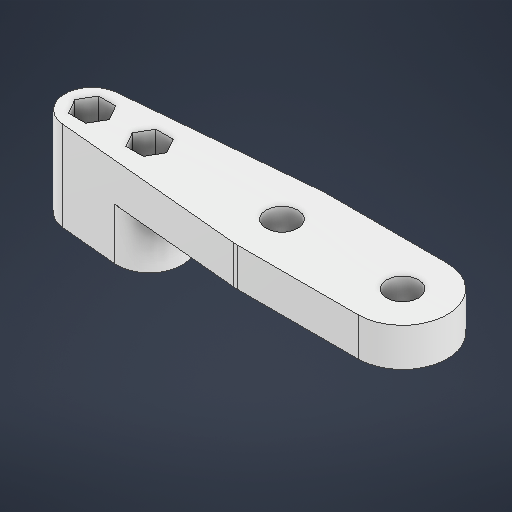
# Autodesk Inventor part: CNC-012-YAxisLimitSwitchMount
Saved by Autodesk Inventor 2026.2 (Build 302298000, 298)
## iProperties
Created: 2026-06-17
Part Number: CNC-012-YAxisLimitSwitchMount
Material: ABS Plastic
Document SubType Name: Modeling
Designer: Kenji
Density: 1.06 g/cm^3
Appearance: Smooth - White
Author: Kenji
Autodesk Inventor part; units mm, degrees
ref_plane "YZ Plane" through (0, 0, 0) normal (1, 0, 0) x (0, 1, 0)
ref_plane "XZ Plane" through (0, 0, 0) normal (0, 1, 0) x (-1, 0, 0)
ref_plane "XY Plane" through (0, 0, 0) normal (0, 0, 1) x (1, 0, 0)
sketch "Sketch1" plane through (0, 0, 0) normal (0, 1, 0) x (-1, 0, 0)
  circle A0 centre (0, 0) radius 1.35
  circle A1 centre (-9.525, 0) radius 1.35
  circle A2 centre (-31.4566, 0) radius 2.63
  circle A3 centre (-51.4566, 0) radius 2.63
  circle A4 centre (0, 0) radius 4.525 construction
  circle A5 centre (-9.525, 0) radius 4.525 construction
  circle A6 centre (-31.4566, 0) radius 7.3925 construction
  circle A7 centre (-51.4566, 0) radius 7.3925 construction
  line L0 (0.4125, 4.5062) -> (-30.7827, 7.3617)
  line L1 (0.4125, -4.5062) -> (-30.7827, -7.3617)
  line L2 (-31.4566, 7.3925) -> (-51.4566, 7.3925)
  line L3 (-31.4566, -7.3925) -> (-51.4566, -7.3925)
  arc A8 (-51.4566, 7.3925) -> (-51.4566, -7.3925) centre (-51.4566, 0) ccw
  arc A9 (-31.4566, -7.3925) -> (-30.7827, -7.3617) centre (-31.4566, 0) ccw
  arc A10 (-30.7827, 7.3617) -> (-31.4566, 7.3925) centre (-31.4566, 0) ccw
  arc A11 (0.4125, -4.5062) -> (0.4125, 4.5062) centre (0, 0) ccw
  dimension "d0" = 2.7
  dimension "d1" = 9.525
  dimension "d2" = 5.26
  dimension "d3" = 21.9316
  dimension "d4" = 20
  dimension "d5" = 3.175
  dimension "d6" = 4.7625
  constraints: 16 point on circle, 12 centre point, 10 tangent, 8 end point, 4 equal radius, 3 coincident, 3 horizontal alignment, 2 concentric, 2 horizontal
  measures "d0" diameter of A0
  measures "d1" distance of point (0, 0) A1.centre
  measures "d2" diameter of A2
  measures "d3" distance of A2.centre A1.centre
  measures "d4" distance of A3.centre A2.centre
  measures "d5" radial gap between concentric circles of A4 A0
  measures "d6" radial gap between concentric circles of A6 A2
extrude "Extrusion1" add sketch "Sketch1" along normal blind 6.35
sketch "Sketch2" plane through (0, 0, 0) normal (0, -1, 0) x (1, 0, 0)
  line L0 (-0.4125, 4.5062) -> (30.7827, 7.3617) projected
  arc A0 (-0.4125, 4.5062) -> (-0.4125, -4.5062) centre (0, 0) ccw projected
  line L1 (30.7827, -7.3617) -> (-0.4125, -4.5062) projected
  arc A1 (30.7827, -7.3617) -> (31.4566, -7.3925) centre (31.4566, 0) ccw projected
  line L2 (51.4566, -7.3925) -> (31.4566, -7.3925) projected
  arc A2 (51.4566, -7.3925) -> (51.4566, 7.3925) centre (51.4566, 0) ccw projected
  line L3 (31.4566, 7.3925) -> (51.4566, 7.3925) projected
  arc A3 (31.4566, 7.3925) -> (30.7827, 7.3617) centre (31.4566, 0) ccw projected
  circle A4 centre (0, 0) radius 1.35 projected
  circle A5 centre (51.4566, 0) radius 2.63 projected
  circle A6 centre (31.4566, 0) radius 2.63 projected
  circle A7 centre (9.525, 0) radius 1.35 projected
  circle A8 centre (9.525, 0) radius 5.3933 construction
  line L4 (-0.4125, 4.5062) -> (30.7827, 7.3617) projected
  arc A9 (9.0334, -5.3708) -> (9.0334, 5.3708) centre (9.525, 0) ccw
  point P0 (9.0334, 5.3708)
  constraints: 4 point on circle, 2 centre point, 2 point on line, 1 coincident, 1 concentric, 1 tangent
extrude "Extrusion2" add sketch "Sketch2" along normal blind 8.5 contours L0 A9 L1 A0
sketch "Sketch3" plane through (0, 6.35, 0) normal (0, 1, 0) x (1, 0, 0)
  circle A0 centre (9.525, 0) radius 1.35 projected
  line L0 (8.0952, -2.4765) -> (6.6654, 0)
  line L1 (6.6654, 0) -> (8.0952, 2.4765)
  line L2 (8.0952, 2.4765) -> (10.9548, 2.4765)
  line L3 (10.9548, 2.4765) -> (12.3846, 0)
  line L4 (12.3846, 0) -> (10.9548, -2.4765)
  line L5 (10.9548, -2.4765) -> (8.0952, -2.4765)
  line L6 (-1.4298, -2.4765) -> (-2.8596, 0)
  line L7 (-2.8596, 0) -> (-1.4298, 2.4765)
  line L8 (-1.4298, 2.4765) -> (1.4298, 2.4765)
  line L9 (1.4298, 2.4765) -> (2.8596, 0)
  line L10 (2.8596, 0) -> (1.4298, -2.4765)
  line L11 (1.4298, -2.4765) -> (-1.4298, -2.4765)
  point P0 (0, 0)
  point P1 (0, 0)
  dimension "d14" = 4.953
  constraints: 24 end point, 2 coincident, 2 horizontal, 1 collinear, 26 other
  measures "d14" distance between parallel lines of L2 L5
extrude "Extrusion3" cut sketch "Sketch3" against normal blind 13.359
body "Solid1"
